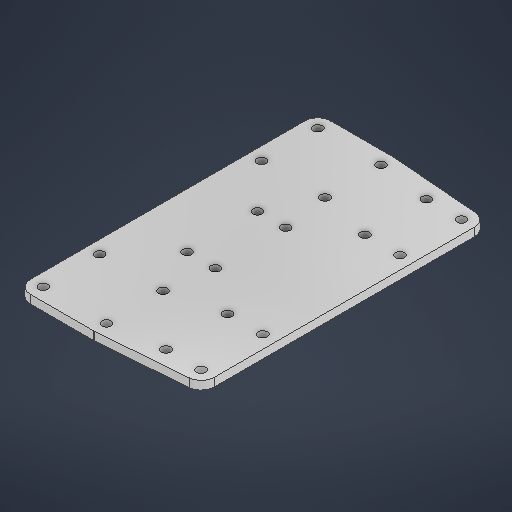
# Autodesk Inventor part: CNC-014-ZAxisSubMount1
Saved by Autodesk Inventor 2026.2 (Build 302298000, 298)
## iProperties
Created: 2026-06-19
Part Number: CNC-014-ZAxisSubMount1
Material: Aluminum 5052
Document SubType Name: Modeling
Designer: Kenji
Mass: 209.663 g
Surface Area: 368.96 cm^2
Volume: 78.2326 cm^3
Density: 2.68 g/cm^3
Appearance: Aluminum - Dark
Author: Kenji
Autodesk Inventor part; units mm, degrees
ref_plane "YZ Plane" through (0, 0, 0) normal (1, 0, 0) x (0, 1, 0)
ref_plane "XZ Plane" through (0, 0, 0) normal (0, 1, 0) x (-1, 0, 0)
sketch "Sketch1" plane through (0, 0, 0) normal (0, 1, 0) x (-1, 0, 0)
  circle A0 centre (0, 0) radius 2.6
  circle A1 centre (-20, 0) radius 2.6
  circle A2 centre (0, 148) radius 2.6
  circle A3 centre (-20, 148) radius 2.6
  circle A4 centre (29.75, -4) radius 2.6
  line L0 (29.75, -4) -> (29.75, -1.4) construction
  line L1 (29.75, -4) -> (32.35, -4) construction
  circle A5 centre (29.75, 28) radius 2.6
  circle A6 centre (65.75, -4) radius 2.6
  circle A7 centre (65.75, 28) radius 2.6
  line L2 (0, 74) -> (-20, 74) construction
  circle A8 centre (26, 54) radius 2.6
  circle A9 centre (42, 54) radius 2.6
  circle A10 centre (26, 94) radius 2.6
  circle A11 centre (42, 94) radius 2.6
  circle A12 centre (29.75, 152) radius 2.6
  circle A13 centre (29.75, 120) radius 2.6
  circle A14 centre (65.75, 152) radius 2.6
  circle A15 centre (65.75, 120) radius 2.6
  circle A16 centre (65.75, -4) radius 7.3625 construction
  circle A17 centre (65.75, 152) radius 7.3625 construction
  circle A18 centre (29.75, 152) radius 7.3625 construction
  circle A19 centre (-20, 148) radius 7.3625 construction
  circle A20 centre (-20, 0) radius 7.3625 construction
  circle A21 centre (29.75, -4) radius 7.3625 construction
  line L3 (73.1125, 152) -> (73.1125, -4)
  line L4 (65.75, -11.3625) -> (29.75, -11.3625)
  line L5 (-20.5901, -7.3388) -> (29.1599, -11.3388)
  line L6 (65.75, 159.3625) -> (29.75, 159.3625)
  line L7 (29.1599, 159.3388) -> (-20.5901, 155.3388)
  line L8 (-27.3625, 148) -> (-27.3625, 0)
  arc A22 (65.75, -11.3625) -> (73.1125, -4) centre (65.75, -4) ccw
  arc A23 (73.1125, 152) -> (65.75, 159.3625) centre (65.75, 152) ccw
  arc A24 (29.75, 159.3625) -> (29.1599, 159.3388) centre (29.75, 152) ccw
  arc A25 (-27.3625, 0) -> (-20.5901, -7.3388) centre (-20, 0) ccw
  arc A26 (-20.5901, 155.3388) -> (-27.3625, 148) centre (-20, 148) ccw
  arc A27 (29.1599, -11.3388) -> (29.75, -11.3625) centre (29.75, -4) ccw
  point P0 (29.75, 30.6)
  point P1 (32.35, 28)
  point P2 (65.75, -1.4)
  point P3 (68.35, -4)
  point P4 (65.75, 30.6)
  point P5 (68.35, 28)
  dimension "d0" = 5.2
  dimension "d1" = 20
  dimension "d2" = 148
  dimension "d3" = 4
  dimension "d4" = 29.75
  dimension "d7" = 32
  dimension "d10" = 36
  dimension "d13" = 74
  dimension "d18" = 16
  dimension "d21" = 40
  dimension "d24" = 20
  dimension "d25" = 26
  dimension "d26" = 4.7625
  constraints: 32 point on circle, 28 centre point, 18 end point, 17 tangent, 12 equal radius, 6 coincident, 4 symmetric about line, 4 vertical alignment, 3 horizontal, 3 vertical, 2 concentric, 2 horizontal alignment, 1 perpendicular, 22 other
  measures "d0" diameter of A0
  measures "d1" distance of A1.centre point (0, 0)
  measures "d2" distance of point (0, 0) A2.centre
  measures "d3" vertical distance of point (0, 0) L0.start
  measures "d4" horizontal distance of point (0, 0) L0.start
  measures "d7" distance of L0.start A5.centre
  measures "d10" distance of L0.start A6.centre
  measures "d13" distance from line of L2 A2.centre
  measures "d18" distance of A8.centre A9.centre
  measures "d21" distance of A8.centre A10.centre
  measures "d24" distance from line of L2 A9.centre
  measures "d25" horizontal distance of point (0, 0) A8.centre
  measures "d26" radial gap between concentric circles of A16 A6
extrude "Extrusion1" add sketch "Sketch1" along normal blind 4.7625
ref_plane "Work Plane1" through (-65.75, 0, 74) normal (0, 0, 1) x (1, 0, 0)
sketch "Sketch3" plane through (0, 4.7625, 0) normal (0, 1, 0) x (1, 0, 0)
  arc A0 (-29.75, -159.3625) -> (-29.1599, -159.3388) centre (-29.75, -152) ccw projected
  line L0 (-29.1599, -159.3388) -> (20.5901, -155.3388) projected
  arc A1 (20.5901, -155.3388) -> (27.3625, -148) centre (20, -148) ccw projected
  line L1 (27.3625, -148) -> (27.3625, 0) projected
  arc A2 (27.3625, 0) -> (20.5901, 7.3388) centre (20, 0) ccw projected
  line L2 (20.5901, 7.3388) -> (-29.1599, 11.3388) projected
  arc A3 (-29.1599, 11.3388) -> (-29.75, 11.3625) centre (-29.75, 4) ccw projected
  line L3 (-29.75, 11.3625) -> (-65.75, 11.3625) projected
  arc A4 (-65.75, 11.3625) -> (-73.1125, 4) centre (-65.75, 4) ccw projected
  line L4 (-73.1125, 4) -> (-73.1125, -152) projected
  arc A5 (-73.1125, -152) -> (-65.75, -159.3625) centre (-65.75, -152) ccw projected
  line L5 (-65.75, -159.3625) -> (-29.75, -159.3625) projected
  circle A6 centre (-29.75, -152) radius 2.6 projected
  circle A7 centre (-65.75, -120) radius 2.6 projected
  circle A8 centre (-26, -94) radius 2.6 projected
  circle A9 centre (-42, -54) radius 2.6 projected
  circle A10 centre (-26, -54) radius 2.6 projected
  circle A11 centre (-65.75, -28) radius 2.6 projected
  circle A12 centre (-29.75, -28) radius 2.6 projected
  circle A13 centre (-29.75, 4) radius 2.6 projected
  circle A14 centre (0, -148) radius 2.6 projected
  circle A15 centre (0, 0) radius 2.6 projected
  circle A16 centre (-42, -94) radius 2.6 projected
  circle A17 centre (-29.75, -120) radius 2.6 projected
  circle A18 centre (-65.75, -152) radius 2.6 projected
  circle A19 centre (-65.75, 4) radius 2.6 projected
  circle A20 centre (20, -148) radius 2.6 projected
  circle A21 centre (20, 0) radius 2.6 projected
  circle A22 centre (0, -113) radius 2.6
  circle A23 centre (20, -113) radius 2.6
  circle A24 centre (0, 0) radius 2.6 projected
  line L6 (-73.1125, -74) -> (27.3625, -74) construction
  line L7 (27.3625, -148) -> (27.3625, 0) construction
  circle A25 centre (0, -35) radius 2.6
  circle A26 centre (20, -35) radius 2.6
  dimension "d56" = 148
  dimension "d60" = 35
  dimension "d61" = 74
  constraints: 4 centre point, 2 end point, 2 equal radius, 2 midpoint, 2 symmetric about line, 2 vertical alignment, 1 horizontal alignment, 1 perpendicular, 2 other
  measures "d56" distance of A1.centre A2.centre
  measures "d60" distance of A1.centre A23.centre
  measures "d61" distance from line of A2.centre L6
extrude "Extrusion3" cut sketch "Sketch3" against normal through all contours A22 | A23
extrude "Extrusion4" cut sketch "Sketch3" against normal through all contours A25 | A26
equation "\"d13\" = 0.5 * d2"
equation "\"d24\" = 0.5 * d21"
body "Solid1"
